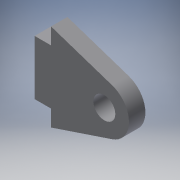
# Autodesk Inventor part: Bearing risers
Saved by Autodesk Inventor 2018 (Build 220112000, 112)
## iProperties
Created: 2018-06-26
Part Number: Bearing risers
Material: Generic
Document SubType Name: Modeling
Designer: Ajith Thomas
Density: 1 g/cm^3
Appearance: Default
Author: Ajith Thomas
Autodesk Inventor part; units mm, degrees
ref_plane "YZ Plane" through (0, 0, 0) normal (1, 0, 0) x (0, 1, 0)
ref_plane "XZ Plane" through (0, 0, 0) normal (0, 1, 0) x (-1, 0, 0)
ref_plane "XY Plane" through (0, 0, 0) normal (0, 0, 1) x (1, 0, 0)
sketch "Sketch1" plane through (0, 0, 0) normal (0, 0, 1) x (1, 0, 0)
  circle A0 centre (0, 0) radius 2 projected
  circle A1 centre (0, 0) radius 3.25 construction
  arc A2 (1.4253, -4.2683) -> (1.4253, 4.2683) centre (0, 0) ccw
  line L0 (0, 0) -> (-9.75, 0) construction
  line L1 (-9.75, 0) -> (-9.75, 8)
  line L2 (-9.75, 8) -> (1.4253, 4.2683)
  line L3 (-9.75, 0) -> (-9.75, -8)
  line L4 (-9.75, -8) -> (1.4253, -4.2683)
  line L5 (-9.75, 5) -> (-12.75, 5)
  line L6 (-12.75, 5) -> (-12.75, -5)
  line L7 (-12.75, -5) -> (-9.75, -5)
  line L8 (-9.75, -5) -> (-9.75, 5)
  point P0 (0, 0)
  point P1 (-9.75, 3)
  dimension "d0" = 9
  dimension "d1" = 9.75
  dimension "d2" = 8
  dimension "d3" = 5
  dimension "d4" = 5
  dimension "d5" = 3
  constraints: 18 end point, 2 horizontal, 2 parallel, 2 point on circle, 2 point on line, 2 symmetric about line, 1 centre point, 1 coincident, 1 perpendicular, 1 tangent, 1 vertical
  measures "d0" diameter of A2
  measures "d1" distance of L0.start L0.end
  measures "d2" distance of L0.end L1.end
  measures "d3" distance between parallel lines of L0 L5
  measures "d4" distance between parallel lines of L0 L7
  measures "d5" distance between parallel lines of L3 L6
extrude "Extrusion2" add sketch "Sketch1" along normal blind 3
body "Solid2"
